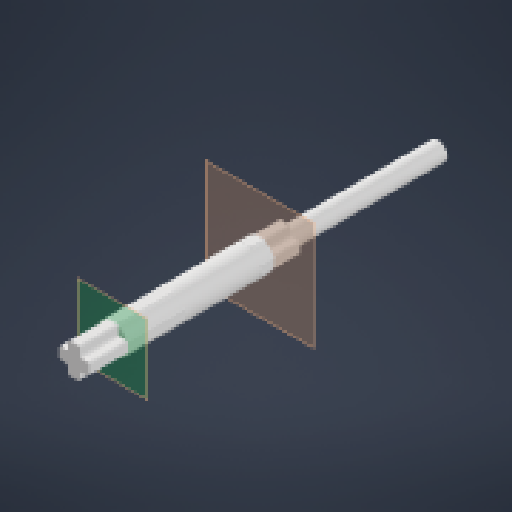
# Autodesk Inventor part: EjeCilintroSuperiorGarra
Saved by Autodesk Inventor 2026.2 (Build 302298010, 298A)
## iProperties
Created: 2026-04-17
Part Number: EjeCilintroSuperiorGarra
Material: Genérico
Document SubType Name: Modeling
Designer: Jose Carlos
Density: 1 g/cm^3
Appearance: Valor por defecto
Author: Jose Carlos
Autodesk Inventor part; units mm, degrees
ref_plane "YZ Plane" through (0, 0, 0) normal (1, 0, 0) x (0, 1, 0)
ref_plane "XZ Plane" through (0, 0, 0) normal (0, 1, 0) x (-1, 0, 0)
ref_plane "XY Plane" through (0, 0, 0) normal (0, 0, 1) x (1, 0, 0)
sketch "Boceto2" plane through (0, 0, 0) normal (0, 0, 1) x (1, 0, 0)
  line L0 (0.9, -6.2636) -> (-0.9, -6.2636)
  line L1 (-0.9, -6.2636) -> (-0.9, -1.4636)
  line L2 (-0.9, -1.4636) -> (0.9, -1.4636)
  line L3 (0.9, -1.4636) -> (0.9, -6.2636)
  line L4 (0.9, -6.2636) -> (-0.9, -1.4636) construction
  line L5 (-0.9, -6.2636) -> (0.9, -1.4636) construction
  line L6 (-2.4, -4.7636) -> (2.4, -4.7636)
  line L7 (2.4, -4.7636) -> (2.4, -2.9636)
  line L8 (2.4, -2.9636) -> (-2.4, -2.9636)
  line L9 (-2.4, -2.9636) -> (-2.4, -4.7636)
  line L10 (-2.4, -4.7636) -> (2.4, -2.9636) construction
  line L11 (2.4, -4.7636) -> (-2.4, -2.9636) construction
  circle A0 centre (0, -3.8636) radius 1.45
  point P0 (0, 0)
  point P1 (1.1369, -2.9636)
  point P2 (0.9, -2.7267)
  point P3 (-0.9, -2.7267)
  point P4 (-1.1369, -2.9636)
  point P5 (-1.1369, -4.7636)
  point P6 (-0.9, -5.0005)
  point P7 (0.9, -5.0005)
  point P8 (1.1369, -4.7636)
  dimension "d0" = 4.8
  dimension "d1" = 1.8
  dimension "d2" = 1.8
  dimension "d3" = 4.8
  dimension "d4" = 2.9
  constraints: 24 end point, 4 midpoint, 4 parallel, 2 coincident, 2 horizontal, 2 perpendicular, 1 centre point, 1 other
  measures "d0" distance of L0.end L1.end
  measures "d1" distance of L1.end L2.end
  measures "d2" distance of L6.end L7.end
  measures "d3" distance of L7.end L8.end
  measures "d4" diameter of A0
extrude "Extrusión1" add sketch "Boceto2" along normal blind 2 and the other way blind 4
sketch "Boceto3" plane through (0, 0, 2) normal (0, 0, 1) x (1, 0, 0)
  arc A0 (-0.9, -2.7267) -> (-1.1369, -2.9636) centre (0, -3.8636) ccw construction
  circle A1 centre (0, -3.8636) radius 1.45
  arc A2 (1.1369, -2.9636) -> (0.9, -2.7267) centre (0, -3.8636) ccw construction
  point P0 (0, 0)
  point P1 (1.0253, -2.8383)
  constraints: 2 point on circle, 1 centre point, 1 coincident
extrude "Extrusión2" add sketch "Boceto3" along normal blind 12 and the other way blind 30
sketch "Boceto4" plane through (0, -3.8636, 14) normal (0, 0, 1) x (1, 0, 0)
  circle A0 centre (0, 0) radius 1.45 construction
  circle A1 centre (0, 0) radius 1.45
  line L0 (-0.9, 2.4) -> (0.9, 2.4) construction
  line L1 (0.9, -2.4) -> (-0.9, -2.4)
  line L2 (-0.9, -2.4) -> (-0.9, 2.4)
  line L3 (-0.9, 2.4) -> (0.9, 2.4)
  line L4 (0.9, 2.4) -> (0.9, -2.4)
  line L5 (0.9, -2.4) -> (-0.9, 2.4) construction
  line L6 (-0.9, -2.4) -> (0.9, 2.4) construction
  line L7 (2.4, 0.9) -> (-2.4, 0.9)
  line L8 (-2.4, 0.9) -> (-2.4, -0.9)
  line L9 (-2.4, -0.9) -> (2.4, -0.9)
  line L10 (2.4, -0.9) -> (2.4, 0.9)
  line L11 (2.4, 0.9) -> (-2.4, -0.9) construction
  line L12 (-2.4, 0.9) -> (2.4, -0.9) construction
  point P0 (1.1369, 0.9)
  point P1 (0.9, 1.1369)
  point P2 (-0.9, 1.1369)
  point P3 (-1.1369, 0.9)
  point P4 (-1.1369, -0.9)
  point P5 (-0.9, -1.1369)
  point P6 (0.9, -1.1369)
  point P7 (1.1369, -0.9)
  constraints: 24 end point, 4 midpoint, 4 parallel, 2 horizontal, 2 perpendicular, 1 centre point, 1 coincident, 1 concentric
extrude "Extrusión3" add sketch "Boceto4" along normal blind 15
chamfer "Chaflán1" distance 0.2 angle 45 16 edges at (0.9, -1.4636, -1) (-0.9, -1.4636, -1) (-2.4, -2.9636, -1) (-2.4, -4.7636, -1) (-0.9, -6.2636, -1) (0.9, -6.2636, -1) (2.4, -4.7636, -1) (2.4, -2.9636, -1) (2.4, -2.9636, 21.5) (0.9, -1.4636, 21.5) (-0.9, -1.4636, 21.5) (-2.4, -2.9636, 21.5) (-2.4, -4.7636, 21.5) (-0.9, -6.2636, 21.5) (0.9, -6.2636, 21.5) (2.4, -4.7636, 21.5)
ref_plane "Plano de trabajo1" through (0, -3.8636, 23) normal (0, 0, -1) x (-1, 0, 0)
sketch "Boceto5" plane through (0, -3.8636, 23) normal (0, 0, -1) x (-1, 0, 0)
  circle A0 centre (0, 0) radius 1.45 construction
  circle A1 centre (0, 0) radius 2.4
  line L0 (0.7, 2.4) -> (-0.7, 2.4) construction
  point P0 (0, 3.8636)
  point P1 (0, 2.4)
  constraints: 1 coincident, 1 midpoint, 1 vertical alignment, 2 other
extrude "Extrusión4" add sketch "Boceto5" along normal blind 3
ref_plane "Plano de trabajo2" through (0, 0, 0) normal (0, 0, 1) x (1, 0, 0)
sketch "Boceto6" plane through (0, 0, 0) normal (0, 0, 1) x (1, 0, 0)
  arc A0 (-0.859, -1.6226) -> (-2.241, -3.0046) centre (0, -3.8636) ccw construction
  circle A1 centre (0, -3.8636) radius 2.4
  line L0 (0.7, -1.4636) -> (-0.7, -1.4636) construction
  point P0 (0, 0)
  point P1 (0, -1.4636)
  constraints: 1 coincident, 1 midpoint, 1 vertical alignment, 2 other
extrude "Extrusión5" add sketch "Boceto6" along normal up to surface (20 mm away)
